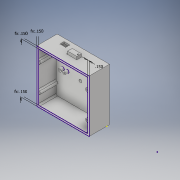
# Autodesk Inventor part: Boxv2
Saved by Autodesk Inventor 2018 (Build 220112000, 112)
## iProperties
Created: 2018-04-19
Part Number: Boxv2
Material: Generic
Document SubType Name: Modeling
Designer: MIABo
Density: 1 g/cm^3
Appearance: Default
Author: MIABo
Autodesk Inventor part; units mm, degrees
note: some values were not read from the file. Chosen so that the rebuilt part matches the saved one: direction of "Hole1".
ref_plane "YZ Plane" through (0, 0, 0) normal (1, 0, 0) x (0, 1, 0)
ref_plane "XZ Plane" through (0, 0, 0) normal (0, 1, 0) x (-1, 0, 0)
ref_plane "XY Plane" through (0, 0, 0) normal (0, 0, 1) x (1, 0, 0)
sketch "Sketch1" plane through (0, 0, 0) normal (0, 0, 1) x (1, 0, 0)
  line L0 (0, 0) -> (-114.3, 0)
  line L1 (-114.3, 0) -> (-114.3, 114.3)
  line L2 (-114.3, 114.3) -> (0, 114.3)
  line L3 (0, 114.3) -> (0, 0)
  dimension "d0" = 114.3
  dimension "d1" = 114.3
  constraints: 8 end point, 2 parallel, 1 horizontal, 1 perpendicular
  measures "d0" distance of L1.end L2.end
  measures "d1" distance of L0.end L1.end
extrude "Extrusion1" add sketch "Sketch1" along normal blind 6.35
sketch "Sketch2" plane through (0, 0, 6.35) normal (0, 0, 1) x (1, 0, 0)
  line L0 (-110.49, 110.49) -> (-3.81, 110.49)
  line L1 (-3.81, 110.49) -> (-3.81, 3.81)
  line L2 (-3.81, 3.81) -> (-110.49, 3.81)
  line L3 (-110.49, 3.81) -> (-110.49, 110.49)
  line L4 (-114.3, 114.3) -> (-114.3, 0) projected
  line L5 (-114.3, 114.3) -> (0, 114.3)
  line L6 (0, 114.3) -> (0, 0)
  line L7 (0, 0) -> (-114.3, 0)
  line L8 (-114.3, 0) -> (-114.3, 114.3)
  dimension "d5" = 3.81
  dimension "d6" = 3.81
  dimension "d7" = 3.81
  dimension "d8" = 3.81
  constraints: 16 end point, 4 parallel, 2 horizontal, 2 perpendicular
  measures "d5" distance between parallel lines of L5 L0
  measures "d6" distance between parallel lines of L6 L1
  measures "d7" distance between parallel lines of L7 L2
  measures "d8" distance between parallel lines of L4 L3
extrude "Extrusion2" add sketch "Sketch2" along normal blind 38.1
sketch "Sketch3" plane through (0, 0, 0) normal (0, 0, -1) x (-1, 0, 0)
  circle A0 centre (109.22, 85.725) radius 3.175
  circle A1 centre (109.22, 28.575) radius 3.175
  line L0 (114.3, 0) -> (114.3, 114.3) projected
  line L1 (114.3, 114.3) -> (0, 114.3) projected
  circle A2 centre (5.08, 85.725) radius 3.175
  circle A3 centre (5.08, 28.575) radius 3.175
  line L2 (0, 114.3) -> (0, 0) projected
  line L3 (0, 0) -> (114.3, 0) projected
  dimension "d11" = 6.35
  dimension "d21" = 57.15
  dimension "d24" = 57.15
  dimension "d25" = 104.14
  dimension "d26" = 104.14
  dimension "d27" = 28.575
  dimension "d29" = 114.3
  dimension "d30" = 5.08
  dimension "d31" = 5.08
  dimension "d32" = 5.08
  constraints: 4 centre point, 3 equal radius
  measures "d11" diameter of A0
  measures "d21" distance of A3.centre A2.centre
  measures "d24" distance of A1.centre A0.centre
  measures "d25" distance of A2.centre A0.centre
  measures "d26" distance of A3.centre A1.centre
  measures "d27" distance from line of L1 A0.centre
  measures "d29" distance of L0.start L0.end
  measures "d30" distance from line of A0.centre L0
  measures "d31" distance from line of L2 A3.centre
  measures "d32" distance from line of L0 A1.centre
extrude "Extrusion3" add sketch "Sketch3" against normal up to surface (44.45 mm away) contours A0 | A1 | A2 | A3
sketch "Sketch4" plane through (0, 0, 0) normal (0, 0, -1) x (-1, 0, 0)
  line L0 (0, 114.3) -> (0, 0) projected
  line L1 (114.3, 114.3) -> (0, 114.3) projected
  point P0 (57.15, 57.15)
  dimension "d35" = 57.15
  dimension "d36" = 57.15
  measures "d35" distance from line of L0 point (57.15, 57.15)
  measures "d36" distance from line of L1 point (57.15, 57.15)
hole "Hole1" at (-57.15, 57.15, 0) direction (0, 0, 1) diameter 6.35 end up to surface
sketch "Sketch6" plane through (-114.3, 114.3, 0) normal (0, 1, 0) x (1, 0, 0)
  line L0 (47.498, -17.145) -> (70.358, -17.145)
  line L1 (70.358, -17.145) -> (70.358, -27.305)
  line L2 (70.358, -27.305) -> (47.498, -27.305)
  line L3 (47.498, -27.305) -> (47.498, -17.145)
  circle A0 centre (67.818, -22.225) radius 1.524
  line L4 (0, 0) -> (0, -44.45) projected
  line L5 (114.3, -44.45) -> (0, -44.45) projected
  point P0 (114.3, 0)
  point P1 (57.15, -22.225)
  dimension "d44" = 22.86
  dimension "d45" = 10.16
  dimension "d46" = 3.048
  dimension "d47" = 5.08
  dimension "d48" = 2.54
  dimension "d49" = 5.08
  dimension "d50" = 9.652
  dimension "d51" = 57.15
  dimension "d52" = 44.45
  dimension "d53" = 22.225
  constraints: 8 end point, 2 parallel, 1 centre point, 1 horizontal, 1 perpendicular
  measures "d44" distance of L1.end L2.end
  measures "d45" distance of L0.end L1.end
  measures "d46" diameter of A0
  measures "d47" distance from line of L2 A0.centre
  measures "d48" distance from line of L1 A0.centre
  measures "d49" distance from line of L2 point (57.15, -22.225)
  measures "d50" distance from line of L3 point (57.15, -22.225)
  measures "d51" distance from line of L4 point (57.15, -22.225)
  measures "d52" distance of L4.start L4.end
  measures "d53" distance from line of L5 point (57.15, -22.225)
extrude "Extrusion4" add sketch "Sketch6" along normal blind 6.35
sketch "Sketch7" plane through (-114.3, 120.65, 0) normal (0, 1, 0) x (1, 0, 0)
  line L0 (47.498, -17.145) -> (47.498, -27.305) projected
  line L1 (70.358, -27.305) -> (47.498, -27.305) projected
  line L2 (47.498, -17.145) -> (50.038, -17.145)
  line L3 (50.038, -17.145) -> (50.038, -27.305)
  line L4 (50.038, -27.305) -> (47.498, -27.305)
  line L5 (47.498, -27.305) -> (47.498, -17.145)
  point P0 (114.3, 0)
  dimension "d56" = 2.54
  constraints: 8 end point, 2 parallel, 1 horizontal, 1 perpendicular, 1 point on line
  measures "d56" distance of L3.end L4.end
extrude "Extrusion5" cut sketch "Sketch7" against normal up to surface (10.16 mm away)
sketch "Sketch13" plane through (0, 0, 0) normal (0, 0, -1) x (-1, 0, 0)
  circle A0 centre (5.08, 85.725) radius 1.651
  circle A1 centre (109.22, 85.725) radius 1.651
  arc A2 (110.49, 88.6349) -> (110.49, 82.8151) centre (109.22, 85.725) ccw projected
  circle A3 centre (5.08, 28.575) radius 1.651
  circle A4 centre (109.22, 28.575) radius 1.651
  arc A5 (3.81, 25.6651) -> (3.81, 31.4849) centre (5.08, 28.575) ccw projected
  arc A6 (110.49, 31.4849) -> (110.49, 25.6651) centre (109.22, 28.575) ccw projected
  arc A7 (3.81, 82.8151) -> (3.81, 88.6349) centre (5.08, 85.725) ccw projected
  point P0 (0, 0)
  dimension "d108" = 3.302
  constraints: 4 centre point, 4 concentric, 3 equal radius
  measures "d108" diameter of A0
extrude "Extrusion14" cut sketch "Sketch13" against normal up to surface (44.45 mm away)
sketch "Sketch14" plane through (0, 0, 6.35) normal (0, 0, 1) x (1, 0, 0)
  line L0 (-79.6925, 110.49) -> (-77.1525, 110.49)
  line L1 (-77.1525, 110.49) -> (-77.1525, 91.44)
  line L2 (-77.1525, 91.44) -> (-79.6925, 91.44)
  line L3 (-79.6925, 91.44) -> (-79.6925, 110.49)
  line L4 (-102.5525, 110.49) -> (-105.0925, 110.49)
  line L5 (-105.0925, 110.49) -> (-105.0925, 91.44)
  line L6 (-105.0925, 91.44) -> (-102.5525, 91.44)
  line L7 (-102.5525, 91.44) -> (-102.5525, 110.49)
  circle A0 centre (-91.1225, 82.55) radius 3.4925
  circle A1 centre (-91.1225, 82.55) radius 1.524
  circle A2 centre (-86.0425, 61.2648) radius 3.4925
  circle A3 centre (-86.0425, 61.2648) radius 1.524
  circle A4 centre (-96.2025, 61.2648) radius 3.4925
  circle A5 centre (-96.2025, 61.2648) radius 1.524
  line L8 (-3.81, 110.49) -> (-110.49, 110.49) projected
  arc A6 (-110.49, 82.8151) -> (-110.49, 88.6349) centre (-109.22, 85.725) ccw projected
  point P0 (0, 0)
  point P1 (110.49, 6.35)
  point P2 (110.49, 6.35)
  point P3 (-6.985, 110.49)
  point P4 (-107.315, 110.49)
  dimension "d51" = 57.15
  dimension "d139" = 2.54
  dimension "d140" = 19.05
  dimension "d141" = 6.985
  dimension "d145" = 3.048
  dimension "d146" = 6.985
  dimension "d147" = 3.048
  dimension "d148" = 6.985
  dimension "d149" = 3.048
  dimension "d150" = 21.2852
  dimension "d151" = 10.16
  dimension "d153" = 5.08
  dimension "d154" = 49.2252
  dimension "d155" = 27.94
  dimension "d156" = 13.97
  dimension "d183" = 104.14
  dimension "d184" = 104.14
  dimension "d185" = 187.6425
  dimension "d186" = 187.6425
  dimension "d187" = 4.1275
  constraints: 16 end point, 6 centre point, 4 parallel, 3 coincident, 2 equal length, 2 horizontal, 2 perpendicular, 1 collinear, 1 horizontal alignment, 1 point on line
  measures "d139" distance of L6.end L5.end
  measures "d140" distance of L5.end L4.end
  measures "d141" diameter of A0
  measures "d145" diameter of A1
  measures "d146" diameter of A2
  measures "d147" diameter of A3
  measures "d148" diameter of A4
  measures "d149" diameter of A5
  measures "d150" vertical distance of A2.centre A0.centre
  measures "d151" distance of A2.centre A4.centre
  measures "d153" horizontal distance of A2.centre A0.centre
  measures "d154" distance from line of A4.centre L4
  measures "d155" distance between parallel lines of L1 L5
  measures "d156" distance from line of A0.centre L5
  measures "d183" distance from line of point (110.49, 6.35) L8
  measures "d184" distance from line of point (110.49, 6.35) L8
  measures "d185" distance from line of point (110.49, 6.35) L1
  measures "d186" distance from line of point (110.49, 6.35) L1
  measures "d187" distance from line of L5 A6.centre
extrude "Extrusion15" add sketch "Sketch14" along normal blind 6.35
fillet "Fillet3" radius 3.175 4 edges at (-110.49, 110.49, 25.4) (-3.81, 110.49, 25.4) (-3.81, 3.81, 25.4) (-110.49, 3.81, 25.4)
fillet "Fillet4" radius 3.175 8 edges at (-110.49, 25.6651, 25.4) (-110.49, 31.4849, 25.4) (-110.49, 82.8151, 25.4) (-110.49, 88.6349, 25.4) (-3.81, 82.8151, 25.4) (-3.81, 88.6349, 25.4) (-3.81, 25.6651, 25.4) (-3.81, 31.4849, 25.4)
sketch "Sketch16" plane through (-102.5525, 110.49, 6.35) normal (0, -1, 0) x (1, 0, 0)
  line L0 (10.16, 9.525) -> (22.86, 9.525)
  line L1 (22.86, 9.525) -> (22.86, 0.635)
  line L2 (22.86, 0.635) -> (10.16, 0.635)
  line L3 (10.16, 0.635) -> (10.16, 9.525)
  line L4 (22.86, 6.35) -> (25.4, 6.35) projected
  point P0 (102.5525, -6.35)
  dimension "d204" = 5.715
  dimension "d205" = 8.89
  dimension "d206" = 12.7
  dimension "d207" = 2.54
  constraints: 8 end point, 2 parallel, 1 horizontal, 1 perpendicular
  measures "d204" distance between parallel lines of L4 L2
  measures "d205" distance of L0.end L1.end
  measures "d206" distance of L0.start L0.end
  measures "d207" distance from line of L4.end L1
extrude "Extrusion18" cut sketch "Sketch16" against normal blind 8.89
sketch "Sketch17" plane through (0, 0, 44.45) normal (0, 0, 1) x (1, 0, 0)
  line L0 (0, 0) -> (-114.3, 0)
  line L1 (-114.3, 0) -> (-114.3, 114.3)
  line L2 (-114.3, 114.3) -> (0, 114.3)
  line L3 (0, 114.3) -> (0, 0)
  line L4 (-3.81, 3.81) -> (-110.49, 3.81)
  line L5 (-110.49, 3.81) -> (-110.49, 110.49)
  line L6 (-110.49, 110.49) -> (-3.81, 110.49)
  line L7 (-3.81, 110.49) -> (-3.81, 3.81)
  dimension "d210" = 3.81
  dimension "d211" = 3.81
  dimension "d212" = 3.81
  dimension "d213" = 3.81
  constraints: 16 end point, 4 parallel, 2 horizontal, 2 perpendicular
  measures "d210" distance between parallel lines of L3 L7
  measures "d211" distance between parallel lines of L1 L5
  measures "d212" distance between parallel lines of L2 L6
  measures "d213" distance between parallel lines of L0 L4
equation "\"d6\" = d5"
equation "\"d7\" = d5"
equation "\"d8\" = d5"
equation "\"d21\" = d24"
equation "\"d26\" = d25"
equation "\"d31\" = d30"
equation "\"d32\" = d30"
equation "\"d53\" = 0.5 * d52"
body "Solid1"
